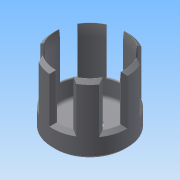
# Autodesk Inventor part: motor_cover
Saved by Autodesk Inventor 2015 (Build 190159000, 159)
## iProperties
Created: 2014-11-23
Part Number: motor_cover
Material: Generic
Document SubType Name: Modeling
Designer: brent
Density: 1 g/cm^3
Appearance: Default
Author: brent
Autodesk Inventor part; units mm, degrees
ref_plane "YZ Plane" through (0, 0, 0) normal (1, 0, 0) x (0, 1, 0)
ref_plane "XZ Plane" through (0, 0, 0) normal (0, 1, 0) x (-1, 0, 0)
sketch "Sketch1" plane through (0, 0, 0) normal (1, 0, 0) x (0, 1, 0)
  line L0 (-14, 0) -> (59.5, 0) projected
  line L1 (0, 0) -> (49, 0)
  line L2 (49, 0) -> (49, -25.3)
  line L3 (49, -25.3) -> (0, -25.3)
  line L4 (0, -25.3) -> (0, 0)
  line L5 (49, -25.3) -> (0, -25.3)
  line L6 (0, -25.3) -> (0, -28.8)
  line L7 (0, -28.8) -> (49, -28.8)
  line L8 (49, -28.8) -> (49, -25.3)
  line L9 (0, -7.5) -> (0, -28.8)
  line L10 (0, -28.8) -> (-3.5, -28.8)
  line L11 (-3.5, -28.8) -> (-3.5, -7.5)
  line L12 (-3.5, -7.5) -> (0, -7.5)
  dimension "d0" = 25.3
  dimension "d1" = 49
  dimension "d2" = 3.5
  dimension "d3" = 7.5
  dimension "d4" = 3.5
  constraints: 24 end point, 6 parallel, 3 perpendicular, 2 collinear, 2 point on line
  measures "d0" distance between parallel lines of L0 L3
  measures "d1" distance between parallel lines of L4 L2
  measures "d2" distance between parallel lines of L3 L7
  measures "d3" distance between parallel lines of L0 L12
  measures "d4" distance between parallel lines of L4 L11
revolve "Revolution1" add sketch "Sketch1" angle 360 about axis through (0, 0, 0) along (0, 1, 0) contours L4 L6 L10 L11 L12 | L8 L7 L6 L3
chamfer "Chamfer1" distance 0.75 angle 45 1 edges at (0, 49, 25.3)
fillet "Fillet1" radius 50.8 1 edges at (0, 48.25, 25.3)
fillet "Fillet2" radius 2.54 1 edges at (0, 0, 25.3)
ref_plane "Work Plane1" through (0, 14, 0) normal (0, 1, 0) x (1, 0, 0)
chamfer "Chamfer2" distance 2.54 angle 45 3 edges at (0, -3.5, 7.5) (0, -3.5, 28.8) (0, 49, 28.8)
sketch "Sketch3" plane through (0, 49, 0) normal (0, 1, 0) x (1, 0, 0)
  circle A0 centre (0, 0) radius 28.8
  line L0 (0, 0) -> (0, 28.8)
  line L1 (0, 0) -> (-12.171406, 26.101664)
  dimension "d17" = 25
  constraints: 4 end point, 2 point on circle, 1 vertical
  measures "d17" angle of L0 L1
extrude "Extrusion2" cut sketch "Sketch3" against normal up to surface (35 mm away) contours L0 L1 A0 picked at (-1.391346, 19.09864)
chamfer "Chamfer3" distance 2.54 angle 45 3 edges at (0, 30.23, -28.8) (-12.1714, 30.23, -26.1017) (-6.2335, 14, -28.1173)
fillet "Fillet3" radius 0.635 1 edges at (-5.4759, 14, -24.7003)
pattern_circular "Circular Pattern1" count 6 over 360 about axis through (0, -1.75, 0) along (0, -1, 0) of "Extrusion2", "Chamfer3", "Fillet3"
body "Solid1"
